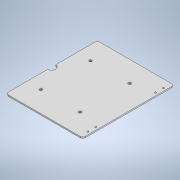
# Autodesk Inventor part: 角度桌板
Saved by Autodesk Inventor 2021 (Build 250183000, 183)
## iProperties
Created: 2023-03-09
Part Number: 角度桌板
Material: 一般
Document SubType Name: Modeling
Designer: brian
Density: 1 g/cm^3
Appearance: 預設
Author: brian
Autodesk Inventor part; units mm, degrees
ref_plane "YZ Plane" through (0, 0, 0) normal (1, 0, 0) x (0, 1, 0)
ref_plane "XZ Plane" through (0, 0, 0) normal (0, 1, 0) x (-1, 0, 0)
ref_plane "XY Plane" through (0, 0, 0) normal (0, 0, 1) x (1, 0, 0)
sketch "草圖1" plane through (0, 0, 0) normal (0, 1, 0) x (-1, 0, 0)
  line L0 (-147, 175) -> (147, 175)
  line L1 (147, 175) -> (147, -175)
  line L2 (147, -175) -> (-147, -175)
  line L3 (-147, -175) -> (-147, 175)
  line L4 (-147, 175) -> (147, -175) construction
  line L5 (147, 175) -> (-147, -175) construction
  point P0 (0, 0)
  dimension "d0" = 294
  dimension "d1" = 350
  constraints: 12 end point, 2 midpoint, 2 parallel, 1 horizontal, 1 perpendicular
  measures "d0" distance of L1.end L2.end
  measures "d1" distance of L0.end L1.end
extrude "擠出1" add sketch "草圖1" along normal blind 5
sketch "草圖2" plane through (0, 5, 0) normal (0, 1, 0) x (1, 0, 0)
  line L0 (147, -175) -> (147, 175) projected
  line L1 (136.5, -114.5) -> (136.5, 114.5) construction
  point P0 (0, 0)
  point P1 (136.5, -144.5)
  point P2 (136.5, 144.5)
  point P3 (136.5, 0)
  point P4 (147, 0)
  dimension "d4" = 30
  dimension "d5" = 30
  dimension "d6" = 10.5
  dimension "d7" = 229
  constraints: 3 vertical alignment, 2 end point, 2 midpoint, 1 horizontal alignment, 1 vertical
  measures "d4" distance of L1.start point (136.5, -144.5)
  measures "d5" distance of point (136.5, 144.5) L1.end
  measures "d6" distance from line of L0 point (136.5, -144.5)
  measures "d7" distance of L1.end L1.start
hole "孔1" at (136.5, 5, 144.5) at (136.5, 5, 114.5) at (136.5, 5, -114.5) at (136.5, 5, -144.5) direction (0, -1, 0) diameter 6 end through all
fillet "圓角1" radius 10 4 edges at (-147, 2.5, 175) (-147, 2.5, -175) (147, 2.5, 175) (147, 2.5, -175)
sketch "草圖4" plane through (0, 5, 0) normal (0, 1, 0) x (1, 0, 0)
  line L0 (-93, -95) -> (57, -95)
  line L1 (57, -95) -> (57, 95)
  line L2 (57, 95) -> (-93, 95)
  line L3 (-93, 95) -> (-93, -95)
  line L4 (-147, 165) -> (-147, -165) projected
  point P0 (0, 0)
  point P1 (-93, 0)
  dimension "d22" = 54
  dimension "d23" = 190
  dimension "d24" = 150
  constraints: 8 end point, 4 coincident, 2 parallel, 1 horizontal, 1 horizontal alignment, 1 midpoint, 1 perpendicular
  measures "d22" distance between parallel lines of L4 L3
  measures "d23" distance of L2.end L0.start
  measures "d24" distance of L0.start L0.end
hole "孔2" at (-93, 5, 95) at (57, 5, 95) at (57, 5, -95) at (-93, 5, -95) direction (0, -1, 0) diameter 10 end through all
sketch "草圖5" plane through (0, 5, 0) normal (0, 1, 0) x (1, 0, 0)
  line L0 (-147, 165) -> (-147, -165) projected
  circle A0 centre (-147, 0) radius 15
  point P0 (0, 0)
  point P1 (-147, 15)
  point P2 (-147, -15)
  dimension "d32" = 30
  constraints: 1 centre point, 1 midpoint
  measures "d32" diameter of A0
extrude "擠出3" cut sketch "草圖5" against normal through all contours A0 L0 picked at (-139.9734, -4.2083)
fillet "圓角3" radius 2 2 edges at (-147, 2.5, 15) (-147, 2.5, -15)
sketch "草圖3" plane through (0, 5, 0) normal (0, 1, 0) x (1, 0, 0)
  arc A0 (-137, 175) -> (-100, 165) centre (-90, 165) ccw projected
  line L0 (-100, 165) -> (-100, -165) projected
  arc A1 (-100, -165) -> (-137, -175) centre (-90, -165) ccw projected
  line L1 (-137, -175) -> (147, -175) projected
  line L2 (100, -175) -> (100, 175) projected
  line L3 (147, 175) -> (-137, 175) projected
  circle A2 centre (89.5, 114.5) radius 3 projected
  circle A3 centre (89.5, -144.5) radius 3 projected
  circle A4 centre (89.5, -114.5) radius 3 projected
  circle A5 centre (89.5, 144.5) radius 3 projected
  line L4 (-137, -175) -> (147, -175) projected
  line L5 (147, 175) -> (-137, 175) projected
  line L6 (147, -175) -> (75, -175)
  line L7 (75, -175) -> (75, 175)
  line L8 (75, 175) -> (100, 175)
  line L9 (100, 175) -> (100, -175)
  line L10 (147, -175) -> (147, 175) projected
  line L11 (75, -154) -> (100, -154)
  line L12 (100, -154) -> (100, -105)
  line L13 (100, -105) -> (75, -105)
  line L14 (75, -105) -> (75, -154)
  line L15 (75, 105) -> (100, 105)
  line L16 (100, 105) -> (100, 154)
  line L17 (100, 154) -> (75, 154)
  line L18 (75, 154) -> (75, 105)
  circle A6 centre (136.5, -144.5) radius 3 construction
  circle A7 centre (136.5, -114.5) radius 3 construction
  line L19 (89.5, -144.5) -> (89.5, -114.5) construction
  circle A8 centre (136.5, 114.5) radius 3 construction
  circle A9 centre (136.5, 144.5) radius 3 construction
  line L20 (89.5, 114.5) -> (89.5, 144.5) construction
  point P0 (0, 0)
  point P1 (100, -129.5)
  point P2 (89.5, -129.5)
  point P3 (100, 129.5)
  point P4 (89.5, 129.5)
  dimension "d16" = 25
  dimension "d17" = 49
  dimension "d18" = 49
  constraints: 22 end point, 5 parallel, 3 horizontal, 3 perpendicular, 3 point on line, 2 horizontal alignment, 2 midpoint, 1 vertical, 17 other
  measures "d16" distance of L7.end L8.end
  measures "d17" distance of L12.end L11.end
  measures "d18" distance of L16.end L15.end
equation "\"d5\" = d4"
